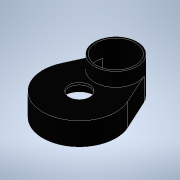
# Autodesk Inventor part: Gear Box Shell
Saved by Autodesk Inventor 2022 (Build 260153000, 153)
## iProperties
Created: 2023-01-26
Part Number: Gear Box Shell
Material: Generic
Document SubType Name: Modeling
Designer: ASUS
Density: 1 g/cm^3
Appearance: Rubber - Black
Author: ASUS
Autodesk Inventor part; units mm, degrees
ref_plane "YZ Plane" through (0, 0, 0) normal (1, 0, 0) x (0, 1, 0)
ref_plane "XZ Plane" through (0, 0, 0) normal (0, 1, 0) x (-1, 0, 0)
ref_plane "XY Plane" through (0, 0, 0) normal (0, 0, 1) x (1, 0, 0)
sketch "Sketch1" plane through (0, 0, 0) normal (0, 1, 0) x (-1, 0, 0)
  circle A0 centre (0, -26.4) radius 7.5 construction
  arc A1 (-12.7268, -32.2333) -> (12.7268, -32.2333) centre (0, -26.4) ccw
  circle A2 centre (0, 0) radius 21.12 construction
  circle A3 centre (0, -26.4) radius 5.28 construction
  line L0 (-22.7265, -10.4167) -> (-12.7268, -32.2333)
  line L1 (22.7265, -10.4167) -> (12.7268, -32.2333)
  arc A4 (22.7265, -10.4167) -> (-22.7265, -10.4167) centre (0, 0) ccw
  arc A5 (-14.0904, -32.8583) -> (14.0904, -32.8583) centre (0, -26.4) ccw
  line L2 (-14.0904, -32.8583) -> (-24.0901, -11.0417)
  arc A6 (24.0901, -11.0417) -> (-24.0901, -11.0417) centre (0, 0) ccw
  line L3 (24.0901, -11.0417) -> (14.0904, -32.8583)
  dimension "d1" = 15
  dimension "d2" = 28
  dimension "d3" = 26.4
  dimension "d4" = 42.24
  dimension "d5" = 10.56
  dimension "d6" = 0
  dimension "d7" = 1.5
  constraints: 8 end point, 8 point on circle, 7 centre point, 4 coincident, 4 tangent, 3 other
  measures "d1" diameter of A0
  measures "d2" diameter of A1
  measures "d3" distance of A0.centre point (0, 0)
  measures "d4" diameter of A2
  measures "d5" diameter of A3
  measures "d6" horizontal distance of A0.centre point (0, 0)
  measures "d7" distance between parallel lines of L1 L3
extrude "Extrusion1" add sketch "Sketch1" along normal blind 1.5 contours L0 A4 L1 A1 | L2 A6 L3 A5
sketch "Sketch2" plane through (0, 0, 0) normal (0, -1, 0) x (1, 0, 0)
  circle A0 centre (0, 0) radius 11.05
  circle A1 centre (0, 0) radius 13
  dimension "d10" = 22.1
  dimension "d11" = 26
  constraints: 2 centre point, 2 coincident
  measures "d10" diameter of A0
  measures "d11" diameter of A1
extrude "Extrusion2" add sketch "Sketch2" along normal blind 7
sketch "Sketch3" plane through (0, 1.5, 0) normal (0, 1, 0) x (1, 0, 0)
  arc A0 (14.0904, 32.8583) -> (-14.0904, 32.8583) centre (0, 26.4) ccw projected
  circle A1 centre (0, 26.4) radius 4.9
  point P0 (0, 0)
  dimension "d14" = 9.8
  constraints: 1 centre point, 1 coincident
  measures "d14" diameter of A1
extrude "Extrusion3" cut sketch "Sketch3" against normal blind 7
sketch "Sketch4" plane through (0, 1.5, 0) normal (0, 1, 0) x (1, 0, 0)
  circle A0 centre (0, 26.4) radius 4.9 projected
  circle A1 centre (0, 26.4) radius 14.125
  circle A2 centre (0, 26.4) radius 15.5
  point P0 (0, 0)
  dimension "d17" = 28.25
  constraints: 2 centre point, 2 coincident
  measures "d17" diameter of A1
extrude "Extrusion4" add sketch "Sketch4" along normal blind 10 contours A2
extrude "Extrusion5" add sketch "Sketch1" against normal blind 15
sketch "Sketch5" plane through (0, 0, 0) normal (0, -1, 0) x (1, 0, 0)
  circle A0 centre (0, 0) radius 7.5
  dimension "d22" = 15
  constraints: 1 centre point, 1 coincident
  measures "d22" diameter of A0
extrude "Extrusion6" cut sketch "Sketch5" against normal blind 15
sketch "Sketch6" plane through (0, 1.5, -26.4) normal (0, 1, 0) x (1, 0, 0)
  circle A0 centre (0, 0) radius 14.125
  point P0 (0, -26.4)
  constraints: 1 centre point
extrude "Extrusion7" cut sketch "Sketch6" against normal blind 15
sketch "Sketch7" plane through (0, 1.5, 0) normal (0, 1, 0) x (1, 0, 0)
  arc A0 (-24.0901, 11.0417) -> (24.0901, 11.0417) centre (0, 0) ccw projected
  line L0 (-26.5, 0) -> (26.5, 0)
  line L1 (26.5, 0) -> (26.5, -144.1644)
  line L2 (26.5, -144.1644) -> (-26.5, -144.1644)
  line L3 (-26.5, -144.1644) -> (-26.5, 0)
  dimension "d27" = 0
  constraints: 8 end point, 2 parallel, 1 horizontal, 1 perpendicular, 1 point on circle
  measures "d27" distance edge to line of A0 L1
body "Solid1"
